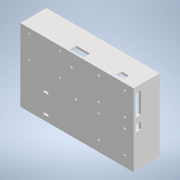
# Autodesk Inventor part: корпус
Saved by Autodesk Inventor 2022 (Build 260153000, 153)
## iProperties
Created: 2023-05-17
Part Number: корпус
Material: Типовые
Document SubType Name: Modeling
Designer: korsh624
Density: 1 g/cm^3
Appearance: По умолчанию
Author: korsh624
Autodesk Inventor part; units mm, degrees
ref_plane "YZ Plane" through (0, 0, 0) normal (1, 0, 0) x (0, 1, 0)
ref_plane "XZ Plane" through (0, 0, 0) normal (0, 1, 0) x (-1, 0, 0)
ref_plane "XY Plane" through (0, 0, 0) normal (0, 0, 1) x (1, 0, 0)
sketch "Эскиз1" plane through (0, 0, 0) normal (0, 0, 1) x (1, 0, 0)
  circle A0 centre (-22.25, 16.75) radius 1.25 projected
  circle A1 centre (22.25, 16.75) radius 1.25 projected
  circle A2 centre (22.25, -16.75) radius 1.25 projected
  circle A3 centre (-22.25, -16.75) radius 1.25 projected
  circle A4 centre (39.25, 4.75) radius 1.6 projected
  circle A5 centre (45.54, -32.2859) radius 1.6 projected
  circle A6 centre (78.75, -19.05) radius 1.5 projected
  circle A7 centre (78.75, 14.55) radius 1.5 projected
  circle A8 centre (116.75, 14.55) radius 1.5 projected
  circle A9 centre (116.75, -19.05) radius 1.5 projected
  circle A10 centre (116.75, -33.45) radius 1.5 projected
  circle A11 centre (78.75, -33.45) radius 1.5 projected
  circle A12 centre (78.75, -67.05) radius 1.5 projected
  circle A13 centre (116.75, -67.05) radius 1.5 projected
  line L0 (-19.75, -46.75) -> (24.25, -46.75) projected
  line L1 (24.25, -71.75) -> (-19.75, -71.75) projected
  line L2 (-1.6455, -46.75) -> (5.3545, -46.75)
  line L3 (5.3545, -46.75) -> (5.3545, -43.75)
  line L4 (5.3545, -43.75) -> (-1.6455, -43.75)
  line L5 (-1.6455, -43.75) -> (-1.6455, -46.75)
  line L6 (-1.6455, -71.75) -> (5.3545, -71.75)
  line L7 (5.3545, -71.75) -> (5.3545, -74.75)
  line L8 (5.3545, -74.75) -> (-1.6455, -74.75)
  line L9 (-1.6455, -74.75) -> (-1.6455, -71.75)
  line L10 (-32.25, 20.55) -> (126.75, 20.55)
  line L11 (126.75, 20.55) -> (126.75, -79.05)
  line L12 (126.75, -79.05) -> (-32.25, -79.05)
  line L13 (-32.25, -79.05) -> (-32.25, 20.55)
  point P0 (0, 0)
  dimension "d0" = 7
  dimension "d1" = 3
  dimension "d2" = 3
  dimension "d3" = 6
  dimension "d4" = 10
  dimension "d5" = 12
  dimension "d6" = 10
  constraints: 24 end point, 6 parallel, 4 point on line, 3 horizontal, 3 perpendicular
  measures "d0" distance of L4.end L3.end
  measures "d1" distance of L3.end L2.end
  measures "d2" distance of L6.end L7.end
  measures "d3" distance from line of L10 A8.centre
  measures "d4" distance from line of A8.centre L11
  measures "d5" distance from line of L12 A13.centre
  measures "d6" distance from line of L13 A3.centre
extrude "Выдавливание1" add sketch "Эскиз1" along normal blind 3
sketch "Эскиз2" plane through (0, 0, 0) normal (0, 0, -1) x (-1, 0, 0)
  line L0 (32.25, 20.55) -> (32.25, -79.05) projected
  line L1 (-126.75, -79.05) -> (-126.75, 20.55) projected
  line L2 (32.25, 20.55) -> (-126.75, 20.55)
  line L3 (-126.75, 20.55) -> (-126.75, -79.05)
  line L4 (-126.75, -79.05) -> (32.25, -79.05)
  line L5 (32.25, -79.05) -> (32.25, 20.55)
  line L6 (35.25, 23.55) -> (-129.75, 23.55)
  line L7 (-129.75, 23.55) -> (-129.75, -82.05)
  line L8 (-129.75, -82.05) -> (35.25, -82.05)
  line L9 (35.25, -82.05) -> (35.25, 23.55)
  point P0 (0, 0)
  point P1 (-126.75, 20.55)
  dimension "d9" = 3
  dimension "d10" = 3
  dimension "d11" = 3
  dimension "d12" = 3
  constraints: 16 end point, 4 parallel, 2 horizontal, 2 perpendicular
  measures "d9" distance between parallel lines of L9 L0
  measures "d10" distance between parallel lines of L1 L7
  measures "d11" distance between parallel lines of L4 L8
  measures "d12" distance between parallel lines of L6 L2
extrude "Выдавливание2" add sketch "Эскиз2" along normal blind 35
sketch "Эскиз3" plane through (0, 0, 0) normal (0, 0, 1) x (1, 0, 0)
  line L0 (129.75, 23.55) -> (129.75, -82.05) projected
  line L1 (-35.25, 23.55) -> (129.75, 23.55) projected
  line L2 (-35.25, -82.05) -> (-35.25, 23.55) projected
  line L3 (129.75, -82.05) -> (-35.25, -82.05) projected
  line L4 (126.75, 20.55) -> (-32.25, 20.55) projected
  line L5 (126.75, -79.05) -> (126.75, 20.55) projected
  line L6 (-32.25, -79.05) -> (126.75, -79.05) projected
  line L7 (-32.25, 20.55) -> (-32.25, -79.05) projected
  point P0 (0, 0)
extrude "Выдавливание3" add sketch "Эскиз3" along normal blind 3
sketch "Эскиз4" plane through (-35.25, 23.55, -35) normal (0, 1, 0) x (1, 0, 0)
  line L0 (82.1894, -30.7775) -> (76.4292, -30.7775) projected
  line L1 (82.1894, -30.7775) -> (76.4292, -30.7775) projected
  line L2 (82.1894, -30.7775) -> (82.3893, -30.7775) projected
  line L3 (3, -35) -> (162, -35) projected
  line L4 (74.4292, -29.1972) -> (84.4292, -29.1972)
  line L5 (84.4292, -29.1972) -> (84.4292, -35)
  line L6 (84.4292, -35) -> (74.4292, -35)
  line L7 (74.4292, -35) -> (74.4292, -29.1972)
  point P0 (35.25, -35)
  dimension "d17" = 10
  dimension "d18" = 2
  constraints: 8 end point, 2 parallel, 1 horizontal, 1 perpendicular, 1 point on line
  measures "d17" distance of L4.start L4.end
  measures "d18" distance from line of L0.end L7
extrude "Выдавливание4" cut sketch "Эскиз4" against normal blind 3
sketch "Эскиз5" plane through (-35.25, 23.55, -35) normal (0, 1, 0) x (1, 0, 0)
  line L0 (74.4292, -35) -> (74.4292, -29.1972) projected
  line L1 (84.4292, -29.1972) -> (84.4292, -35) projected
  line L2 (74.4292, -29.1972) -> (84.4292, -29.1972) projected
  line L3 (84.4292, -35) -> (74.4292, -35) projected
  line L4 (69.2946, -35.2061) -> (89.2946, -35.2061)
  line L5 (89.2946, -35.2061) -> (89.2946, -25.902)
  line L6 (89.2946, -25.902) -> (69.2946, -25.902)
  line L7 (69.2946, -25.902) -> (69.2946, -35.2061)
  point P0 (35.25, -35)
  dimension "d21" = 20
  constraints: 8 end point, 2 parallel, 1 horizontal, 1 perpendicular
  measures "d21" distance of L5.end L6.end
extrude "Выдавливание5" cut sketch "Эскиз5" against normal blind 3
sketch "Эскиз6" plane through (-35.25, 23.55, -35) normal (0, 1, 0) x (1, 0, 0)
  line L0 (135, -33.5) -> (145.5, -33.5) projected
  line L1 (135, -33.5) -> (145.5, -33.5) projected
  line L2 (145.5, -25.5) -> (135, -25.5) projected
  line L3 (135, -33.5) -> (145.5, -33.5)
  line L4 (145.5, -33.5) -> (145.5, -25.5)
  line L5 (145.5, -25.5) -> (135, -25.5)
  line L6 (135, -25.5) -> (135, -33.5)
  point P0 (35.25, -35)
  constraints: 8 end point, 2 parallel, 1 horizontal, 1 perpendicular
extrude "Выдавливание6" cut sketch "Эскиз6" against normal blind 3
sketch "Эскиз7" plane through (129.75, -82.05, -35) normal (1, 0, 0) x (0, 0, -1)
  line L0 (-27.42, 97.05) -> (-27.42, 67.05) projected
  line L1 (-35, 3) -> (-35, 102.6) projected
  line L2 (-35, 97.55) -> (-35, 100.05) projected
  line L3 (-27.42, 67.05) -> (-35, 67.05)
  line L4 (-35, 67.05) -> (-35, 97.55)
  line L5 (-35, 97.55) -> (-27.42, 97.55)
  line L6 (-27.42, 97.55) -> (-27.42, 67.05)
  line L7 (-33.5, 58.3) -> (-22.5, 58.3) projected
  line L8 (-35, 102.6) -> (-35, 3) projected
  line L9 (-27.42, 58.3) -> (-35, 58.3)
  line L10 (-35, 58.3) -> (-35, 48.4289)
  line L11 (-35, 48.4289) -> (-27.42, 48.4289)
  line L12 (-27.42, 48.4289) -> (-27.42, 58.3)
  point P0 (-35, 82.05)
  point P1 (-33.5, 58.3)
  point P2 (-35, 58.3)
  point P3 (-35, 48.4289)
  point P4 (-27.42, 97.05)
  point P5 (-35, 67.05)
  constraints: 16 end point, 4 parallel, 2 horizontal, 2 perpendicular, 2 point on line
extrude "Выдавливание7" cut sketch "Эскиз7" against normal blind 3
sketch "Эскиз8" plane through (-35.25, -82.05, -35) normal (0, -1, 0) x (1, 0, 0)
  line L0 (131, 33.5) -> (131, 22.5) projected
  line L1 (120.5, 33.5) -> (120.5, 22.5) projected
  line L2 (120.5, 22.5) -> (131, 22.5)
  line L3 (131, 22.5) -> (131, 33.5)
  line L4 (131, 33.5) -> (120.5, 33.5)
  line L5 (120.5, 33.5) -> (120.5, 22.5)
  point P0 (35.25, 35)
  constraints: 8 end point, 2 parallel, 1 horizontal, 1 perpendicular
extrude "Выдавливание8" cut sketch "Эскиз8" against normal blind 3
sketch "Эскиз9" plane through (-35.25, -82.05, -35) normal (-1, 0, 0) x (0, 0, 1)
  line L0 (23.42, 97.05) -> (23.42, 67.05) projected
  line L1 (33.67, 64.8) -> (33.67, 99.3) projected
  line L2 (35, 67.05) -> (27.42, 67.05) projected
  line L3 (23.42, 97.05) -> (33.67, 97.05)
  line L4 (33.67, 97.05) -> (33.67, 67.05)
  line L5 (33.67, 67.05) -> (23.42, 67.05)
  line L6 (23.42, 67.05) -> (23.42, 97.05)
  point P0 (35, 82.05)
  point P1 (23.42, 67.05)
  point P2 (27.42, 67.05)
  constraints: 8 end point, 2 parallel, 2 point on line, 1 horizontal, 1 perpendicular
extrude "Выдавливание9" cut sketch "Эскиз9" against normal blind 3
